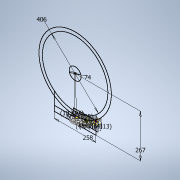
# Autodesk Inventor part: ArrayBracket
Saved by Autodesk Inventor 2022 (Build 260153070, 153G)
## iProperties
Created: 2021-11-12
Part Number: ArrayBracket
Material: Generic
Document SubType Name: Modeling
Designer: elmar
Density: 1 g/cm^3
Appearance: Default
Author: elmar
Autodesk Inventor part; units mm, degrees
ref_plane "YZ Plane" through (0, 0, 0) normal (1, 0, 0) x (0, 1, 0)
ref_plane "XZ Plane" through (0, 0, 0) normal (0, 1, 0) x (-1, 0, 0)
ref_plane "XY Plane" through (0, 0, 0) normal (0, 0, 1) x (1, 0, 0)
sketch "Sketch1" plane through (0, 0, 0) normal (0, 0, 1) x (1, 0, 0)
  circle A0 centre (0, 0) radius 203
  line L0 (-129, -156.7418) -> (-129, -267)
  line L1 (-129, -267) -> (129, -267)
  line L2 (129, -267) -> (129, -156.7418)
  circle A1 centre (0, 0) radius 37
  line L3 (0, -203) -> (0, -267)
  line L4 (0, -235) -> (-129, -235)
  line L5 (0, -235) -> (11.5, -235)
  dimension "d0" = 406
  dimension "d1" = 267
  dimension "d2" = 74
  dimension "d3" = 258
  dimension "d11" = 11.5
  dimension "HalfAngle" = 2.802
  constraints: 12 end point, 3 perpendicular, 3 point on circle, 2 centre point, 2 coincident, 2 midpoint, 2 vertical, 1 horizontal, 1 parallel, 1 point on line
  measures "d0" diameter of A0
  measures "d1" distance from line of L1 point (0, 0)
  measures "d2" diameter of A1
  measures "d3" distance of L0.end L1.end
  measures "d11" distance of L4.start L5.end
extrude "Extrusion1" add sketch "Sketch1" along normal blind 74 contours A1
ref_plane "Work Plane1" through (0, -235, 0) normal (0, -1, 0) x (-1, 0, 0)
sketch "Sketch2" plane through (0, -235, 0) normal (0, -1, 0) x (-1, 0, 0)
  line L0 (0, 13.2791) -> (11.5, 6.6395)
  line L1 (11.5, 6.6395) -> (11.5, -6.6395)
  line L2 (11.5, -6.6395) -> (0, -13.2791)
  line L3 (0, -13.2791) -> (-11.5, -6.6395)
  line L4 (-11.5, -6.6395) -> (-11.5, 6.6395)
  line L5 (-11.5, 6.6395) -> (0, 13.2791)
  point P0 (0, 0)
  point P1 (0, 0)
  dimension "d8" = 23
  constraints: 12 end point, 1 coincident, 1 vertical, 13 other
  measures "d8" distance between parallel lines of L1 L4
extrude "Extrusion2" add sketch "Sketch2" along normal blind 2 draft 2.802 separate body
sketch "Sketch3" plane through (0, -235, 0) normal (0, 1, 0) x (1, 0, 0)
  line L0 (0, 0) -> (-5.7989, -10.0441)
  line L1 (-11.5979, -6.696) -> (0, -13.3921) projected
  point P0 (-0.635, -1.0999)
  point P1 (-1.905, -3.2996)
  point P2 (-3.175, -5.4993)
  dimension "d16" = 1.27
  dimension "d17" = 2.54
  dimension "d18" = 2.54
  constraints: 3 point on line, 2 end point, 1 midpoint
  measures "d16" distance of L0.start point (-0.635, -1.1)
  measures "d17" distance of point (-0.635, -1.1) point (-1.905, -3.3)
  measures "d18" distance of point (-1.905, -3.3) point (-3.175, -5.499)
hole "Hole1" at (-1.905, -235, 3.2996) at (-0.635, -235, 1.0999) at (-3.175, -235, 5.4993) direction (0, -1, 0) diameter 0.7165 end through all bodies 2
pattern_circular "Circular Pattern1" count 7 over 33.619 about axis through (0, 0, -10) along (0, 0, 1) of "Extrusion2", "Hole1" bodies 2 skipped copies 4
ref_plane "Work Plane2" through (0, -235, -13.2791) normal (-0.0487035, 0.9952446, 0.0843569) x (0.8660254, 0, 0.5)
sketch "Sketch4" plane through (0, -235, -13.2791) normal (-0.0487035, 0.9952446, 0.0843569) x (0.8660254, 0, 0.5)
  line L0 (-0.0475, 22.9725) -> (13.2157, 22.9999)
  line L1 (13.2157, 22.9999) -> (19.871, 11.5273)
  line L2 (19.871, 11.5273) -> (13.2632, 0.0274)
  line L3 (13.2632, 0.0274) -> (0, 0)
  line L4 (0, 0) -> (-6.6553, 11.4725)
  line L5 (-6.6553, 11.4725) -> (-0.0475, 22.9725)
  point P0 (6.6395, 11.4453)
  point P1 (6.6078, 11.4999)
  point P2 (0, 0)
  constraints: 12 end point, 2 coincident, 13 other
extrude "Extrusion3" add sketch "Sketch4" against normal blind 2 draft 2.802 separate body
sketch "Sketch5" plane through (0, -235, -13.2791) normal (-0.0487035, 0.9952446, 0.0843569) x (0.8660254, 0, 0.5)
  line L0 (6.6395, 11.4453) -> (6.6316, 0.0137)
  line L1 (0, 0) -> (13.2632, 0.0274) projected
  point P0 (6.6386, 10.1753)
  point P1 (6.6369, 7.6353)
  point P2 (6.6351, 5.0953)
  dimension "d28" = 1.27
  dimension "d29" = 2.54
  dimension "d30" = 2.54
  constraints: 3 point on line, 2 end point, 1 midpoint
  measures "d28" distance of point (6.639, 10.175) L0.start
  measures "d29" distance of point (6.637, 7.635) point (6.639, 10.175)
  measures "d30" distance of point (6.635, 5.095) point (6.637, 7.635)
hole "Hole2" at (10.8127, -234.0089, -18.7299) at (9.5472, -234.2563, -16.5415) at (8.2817, -234.5037, -14.3532) direction (0.0487035, -0.9952446, -0.0843569) diameter 0.7165 end through all bodies 3
pattern_circular "Circular Pattern2" count 6 over 28.016 about axis through (0, 0, -10) along (0, 0, 1) of "Extrusion3", "Hole2" bodies 3
mirror "Mirror1" about plane through (0, 0, 0) normal (0, 0, 1) of "Extrusion3", "Hole2", "Circular Pattern2" bodies 3
ref_plane "Work Plane3" through (120.4045, -201.8394, -33.3842) normal (0, 0, 1) x (-0.957271, -0.2891923, 0)
sketch "Sketch6" plane through (120.4045, -201.8394, -33.3842) normal (0, 0, 1) x (-0.957271, -0.2891923, 0)
  line L0 (0, 0) -> (11.0499, 3.3354) projected
  line L1 (11.0499, 3.3354) -> (22.5368, 4.465) projected
  line L2 (10.9946, 3.33) -> (11.0499, 3.3354) projected
  line L3 (22.5368, 4.465) -> (33.8596, 6.7056) projected
  line L4 (33.8596, 6.7056) -> (45.4019, 6.7083) projected
  line L5 (45.4019, 6.7083) -> (56.8894, 7.8326) projected
  line L6 (56.8894, 7.8326) -> (68.3768, 6.7083) projected
  line L7 (68.3768, 6.7083) -> (79.9191, 6.7056) projected
  line L8 (79.9191, 6.7056) -> (91.2419, 4.465) projected
  line L9 (91.2419, 4.465) -> (102.7288, 3.3354) projected
  line L10 (102.7288, 3.3354) -> (113.7787, 0) projected
  arc A0 (127.4729, 5.4101) -> (-13.6942, 5.4101) centre (56.8894, -228.035) ccw
  line L11 (-10.8, -4.1619) -> (-13.6942, 5.4101)
  line L12 (127.4729, 5.4101) -> (124.5787, -4.1619)
  line L13 (-10.8, -4.1619) -> (0.4801, -1.9244) projected
  line L14 (0.4801, -1.9244) -> (11.4367, 1.3829) projected
  line L15 (11.4367, 1.3829) -> (22.8267, 2.503) projected
  line L16 (22.8267, 2.503) -> (34.0539, 4.7246) projected
  line L17 (34.0539, 4.7246) -> (45.4989, 4.7273) projected
  line L18 (45.4989, 4.7273) -> (56.8894, 5.8421) projected
  line L19 (56.8894, 5.8421) -> (68.2799, 4.7273) projected
  line L20 (68.2799, 4.7273) -> (79.7248, 4.7246) projected
  line L21 (79.7248, 4.7246) -> (90.952, 2.503) projected
  line L22 (90.952, 2.503) -> (102.342, 1.3829) projected
  line L23 (102.342, 1.3829) -> (113.2986, -1.9244) projected
  line L24 (113.2986, -1.9244) -> (124.5787, -4.1619) projected
  dimension "d79" = 10
  constraints: 4 end point, 2 point on circle, 2 point on line, 1 centre point, 1 coincident
  measures "d79" distance of L11.start L11.end
extrude "Extrusion4" add sketch "Sketch6" along normal blind 10 separate body
fillet "Fillet1" radius 9 3 edges at (135.0781, -203.0581, -28.3842) (70.5289, -233.4617, -23.3842) (-0.057, -243.8825, -28.3842)
mirror "Mirror2" about plane through (0, 0, 0) normal (0, 0, 1) of "Extrusion4", "Fillet1" bodies 4
ref_plane "Work Plane4" through (79.6409, -223.5192, 6.6395) normal (0.2891923, -0.957271, 0) x (0, 0, 1)
ref_plane "Work Plane5" through (70.5289, -233.4617, 33.3842) normal (0.2891923, -0.957271, 0) x (0.957271, 0.2891923, 0)
sketch "Sketch7" plane through (70.5289, -233.4617, 33.3842) normal (0.2891923, -0.957271, 0) x (0.957271, 0.2891923, 0)
  line L0 (-11.5979, -26.6882) -> (-11.5979, -40.0803) projected
  line L1 (11.5979, -40.0803) -> (11.5979, -26.6882) projected
  line L2 (61.5868, -65.7685) -> (-61.5868, -65.7685) projected
  line L3 (61.5868, -1) -> (-61.5868, -1) projected
  line L4 (5, -1) -> (-5, -1)
  line L5 (-5, -1) -> (-5, -65.7685)
  line L6 (-5, -65.7685) -> (5, -65.7685)
  line L7 (5, -65.7685) -> (5, -1)
  line L8 (5, -1) -> (-5, -65.7685) construction
  line L9 (-5, -1) -> (5, -65.7685) construction
  line L10 (12.7, -24.4942) -> (-12.7, -24.4942)
  line L11 (-12.7, -24.4942) -> (-12.7, -42.2742)
  line L12 (-12.7, -42.2742) -> (12.7, -42.2742)
  line L13 (12.7, -42.2742) -> (12.7, -24.4942)
  line L14 (12.7, -24.4942) -> (-12.7, -42.2742) construction
  line L15 (-12.7, -24.4942) -> (12.7, -42.2742) construction
  circle A0 centre (0, -33.3842) radius 6.015
  line L16 (10.16, -27.0342) -> (-10.16, -27.0342)
  line L17 (-10.16, -27.0342) -> (-10.16, -39.7342)
  line L18 (-10.16, -39.7342) -> (10.16, -39.7342)
  line L19 (10.16, -39.7342) -> (10.16, -27.0342)
  line L20 (10.16, -27.0342) -> (-10.16, -39.7342) construction
  line L21 (-10.16, -27.0342) -> (10.16, -39.7342) construction
  line L22 (0, -88.2453) -> (0, 62.0926) projected
  point P0 (0, -33.3842)
  point P1 (0, -27.0342)
  point P2 (-5, -24.4942)
  point P3 (-5, -42.2742)
  point P4 (5, -42.2742)
  point P5 (5, -24.4942)
  point P6 (5, -1)
  point P7 (-5, -1)
  dimension "d45" = 10
  dimension "d46" = 12.03
  dimension "d47" = 25.4
  dimension "d48" = 17.78
  dimension "d49" = 12.7
  dimension "d50" = 20.32
  dimension "d51" = 2.54
  constraints: 36 end point, 6 midpoint, 6 parallel, 3 horizontal, 3 perpendicular, 2 point on line, 1 centre point, 1 coincident
  measures "d45" distance between parallel lines of L7 L5
  measures "d46" diameter of A0
  measures "d47" distance of L11.end L12.end
  measures "d48" distance of L10.end L11.end
  measures "d49" distance of L18.end L16.start
  measures "d50" distance of L16.start L16.end
  measures "d51" distance from line of point (0, -27.034) L10
extrude "Extrusion5" add sketch "Sketch7" against normal blind 2 contours L2 L22 L12 L7 | L2 L5 L12 L22 | L12 L22 L18 L7 | L7 L18 L19 L16 L10 L13 L12 | L12 L5 L18 L22 | L18 L22 A0 L7 | L7 A0 L16 L19 L18 | L12 L11 L10 L5 L16 L17 L18 | L18 L5 A0 L22 | L18 L17 L16 L5 A0 | A0 L22 L16 L7 | L10 L22 L3 L7 | L7 L16 L22 L10 | A0 L5 L16 L22 | L22 L16 L5 L10 | L10 L5 L3 L22 bodies 4
hole "Hole3" at (70.5289, -233.4617, 6.35) direction (-0.2891923, 0.957271, 0) diameter 0.7165 depth 2 tip angle 118 bodies 4
pattern_linear "Rectangular Pattern1" count 5 spacing 2.54 along (-0.957271, -0.2891923, 0) of "Hole3" first direction both ways yes bodies 4
hole "Hole4" at (60.8031, -236.3998, -6.35) at (60.8031, -236.3998, 6.35) at (80.2548, -230.5235, 6.35) at (80.2548, -230.5235, -6.35) direction (-0.2891923, 0.957271, 0) diameter 2.5 depth 2 tip angle 118 bodies 4
sketch "Sketch8" plane through (0, 0, 0) normal (0, 0, 1) x (1, 0, 0)
  line L0 (-11.5979, -189.3257) -> (140.8779, -189.3257)
  line L1 (140.8779, -189.3257) -> (140.8779, -243.7121)
  line L2 (140.8779, -243.7121) -> (-11.5979, -243.7121)
  line L3 (-11.5979, -243.7121) -> (-11.5979, -189.3257)
  line L4 (-11.5979, -189.3257) -> (140.8779, -243.7121) construction
  line L5 (140.8779, -189.3257) -> (-11.5979, -243.7121) construction
  arc A0 (-0.0549, -234.71) -> (9.2879, -243.7056) centre (8.9451, -234.7121) ccw projected
  arc A1 (127.1983, -208.0847) -> (129.9978, -195.421) centre (122.5043, -200.4058) ccw projected
  line L6 (-0.0547, -233.8825) -> (-0.0549, -234.71) projected
  arc A2 (9.2879, -243.7056) -> (127.1983, -208.0847) centre (0, 0) ccw projected
  line L7 (129.9978, -195.421) -> (129.5395, -194.732) projected
  line L8 (68.5386, -226.8733) -> (67.9602, -224.9587) projected
  line L9 (68.5386, -226.8733) -> (69.9506, -231.5471)
  line L10 (69.6076, -231.6507) -> (70.2935, -231.4435) projected
  point P0 (0, 0)
  point P1 (64.64, -216.5189)
  point P2 (-11.5979, -237)
  point P3 (140.8779, -190.9369)
  point P4 (139.6891, -189.3257)
  point P5 (-0.0553, -235.873)
  point P6 (130.642, -196.3893)
  point P7 (70.0689, -231.5114)
  point P8 (69.8323, -231.5829)
  point P9 (69.2446, -229.2102)
  dimension "d71" = 57.8643
  dimension "d72" = 55.6949
  dimension "d73" = 18.1932
  dimension "d74" = 16.1131
  dimension "d75" = 4.6045
  dimension "d76" = 12.6913
  constraints: 14 end point, 4 midpoint, 3 point on line, 2 parallel, 1 horizontal, 1 perpendicular, 1 tangent
  measures "d71" horizontal distance of A1.centre point (64.64, -216.519)
  measures "d72" horizontal distance of A0.centre point (64.64, -216.519)
  measures "d73" vertical distance of A0.centre point (64.64, -216.519)
  measures "d74" vertical distance of A1.centre point (64.64, -216.519)
  measures "d75" horizontal distance of point (64.64, -216.519) point (69.245, -229.21)
  measures "d76" vertical distance of point (64.64, -216.519) point (69.245, -229.21)
sketch "Sketch9" plane through (0, 0, 0) normal (0, 0, 1) x (1, 0, 0)
  circle A0 centre (0, 0) radius 224.2409
  line L0 (78.2169, -219.5226) -> (67.6355, -223.8838) projected
  line L1 (78.2169, -219.5226) -> (75.2633, -211.2331)
  line L2 (99.277, -210.8367) -> (89.172, -216.2103) projected
  line L3 (89.172, -216.2103) -> (85.4979, -207.3019)
  line L4 (67.6355, -223.8838) -> (56.4093, -226.1107) projected
  line L5 (67.6355, -223.8838) -> (64.8487, -214.6593)
  dimension "d77" = 8.8
  dimension "d78" = 21.9208
  constraints: 6 end point, 3 line through centre, 3 point on circle, 1 centre point, 1 coincident
  measures "d77" distance of L0.start L1.end
  measures "d78" distance of L5.end L3.end
sketch "Sketch10" plane through (119.3884, -200.1361, 33.1029) normal (-0.5104808, 0.8557414, -0.0843569) x (0.7653531, 0.4074478, -0.4982178)
  circle A0 centre (6.6526, 15.3509) radius 0.3583 projected
  circle A1 centre (6.6456, 17.8909) radius 0.3583 projected
  circle A2 centre (6.6597, 12.8109) radius 0.3583 projected
  line L0 (0, 22.9725) -> (-6.5999, 11.4314) projected
  line L1 (0, 0) -> (-6.5999, 11.4314) projected
  line L2 (13.2632, 0) -> (0, 0) projected
  line L3 (19.8948, 11.4863) -> (13.2632, 0) projected
  line L4 (13.2632, 22.9725) -> (19.8948, 11.4863) projected
  line L5 (0, 22.9725) -> (13.2632, 22.9725) projected
  point P0 (6.6632, 11.5409)
extrude "Extrusion6" cut sketch "Sketch10" along normal blind 10 bodies 3 4
pattern_circular "Circular Pattern3" count 6 over 28.016 about axis through (0, 0, -10) along (0, 0, -1) of "Extrusion6" bodies 4
mirror "Mirror3" about plane through (0, 0, 0) normal (0, 0, 1) of "Extrusion6", "Circular Pattern3" bodies 4
equation "\"d11\" = 0.5 * d8"
equation "\"d10\" = HalfAngle"
equation "\"d14\" = 12 * HalfAngle"
equation "\"d27\" = HalfAngle"
equation "\"d39\" = 10 * HalfAngle"
equation "\"d83\" = 10 * HalfAngle"
body "Solid1"
body "Solid2"
body "Solid3"
body "Solid4"
